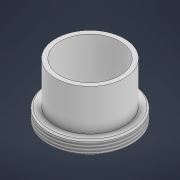
# Autodesk Inventor part: 018
Saved by Autodesk Inventor 2022 (Build 260153000, 153)
## iProperties
Created: 2021-11-15
Part Number: 018
Material: Generic
Document SubType Name: Modeling
Designer: vinicius.miguel
Density: 1 g/cm^3
Appearance: Default
Author: vinicius.miguel
Autodesk Inventor part; units mm, degrees
ref_plane "YZ Plane" through (0, 0, 0) normal (1, 0, 0) x (0, 1, 0)
ref_plane "XZ Plane" through (0, 0, 0) normal (0, 1, 0) x (-1, 0, 0)
ref_plane "XY Plane" through (0, 0, 0) normal (0, 0, 1) x (1, 0, 0)
sketch "Sketch1" plane through (0, 0, 0) normal (0, 0, 1) x (1, 0, 0)
  line L0 (0, 0) -> (0, 18.35)
  line L1 (12, 0) -> (12, 3)
  line L2 (12, 3) -> (10, 3)
  line L3 (10, 3) -> (10, 18.35)
  line L4 (10, 18.35) -> (11.5, 18.35)
  line L5 (11.5, 18.35) -> (11.5, 4.5)
  line L6 (11.5, 4.5) -> (14, 4.5)
  line L7 (14, 4.5) -> (14, 0)
  line L8 (14, 0) -> (12, 0)
  dimension "d0" = 24
  dimension "d1" = 2
  dimension "d2" = 1.5
  dimension "d3" = 1.5
  dimension "d4" = 4.5
  dimension "d5" = 20
  dimension "d7" = 18.35
  constraints: 18 end point, 7 perpendicular, 2 horizontal alignment, 2 vertical
  measures "d0" diameter of L1 L0
  measures "d1" distance of L7.end L1.start
  measures "d2" distance between parallel lines of L5 L3
  measures "d3" distance between parallel lines of L6 L2
  measures "d4" distance between parallel lines of L6 L8
  measures "d5" diameter of L3 L0
  measures "d7" distance from line of L0.start L4
revolve "Revolution1" add sketch "Sketch1" angle 360 about axis through (0, 0, 0) along (0, 1, 0)
chamfer "Chamfer1" distance 0.5 angle 45 2 edges at (-14, 4.5, 0) (-14, 0, 0)
thread "Thread1" size "M28x1" class "6g" standard "ANSI Metric M Profile" full length
equation "\"d3\" = d2"
body "Solid1"
